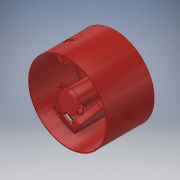
# Autodesk Inventor part: BottomPlatform
Saved by Autodesk Inventor 2019 (Build 230136000, 136)
## iProperties
Created: 2022-07-06
Part Number: BottomPlatform
Material: Generic
Document SubType Name: Modeling
Designer: zreik
Density: 1 g/cm^3
Appearance: Orange-Red
d104: 190.000 mm
Author: zreik
Autodesk Inventor part; units mm, degrees
ref_plane "XZ Plane" through (0, 0, 0) normal (0, 1, 0) x (-1, 0, 0)
ref_plane "XY Plane" through (0, 0, 0) normal (0, 0, 1) x (1, 0, 0)
sketch "Sketch1" plane through (0, 0, 0) normal (0, 0, 1) x (1, 0, 0)
  circle A0 centre (0, 0) radius 25
  line L0 (15, -5) -> (35, -5)
  line L1 (35, -5) -> (35, 5)
  line L2 (35, 5) -> (15, 5)
  line L3 (15, 5) -> (15, -5)
  line L4 (15, -5) -> (35, 5) construction
  line L5 (35, -5) -> (15, 5) construction
  point P0 (25, 0)
  dimension "d0" = 50
  dimension "d3" = 10
  dimension "d4" = 20
  dimension "d5" = 0
  constraints: 12 end point, 2 midpoint, 2 parallel, 1 coincident, 1 horizontal, 1 horizontal alignment, 1 perpendicular, 2 other
  measures "d3" distance of L0.end L1.end
  measures "d4" distance of L0.start L0.end
  measures "d5" vertical distance of point (0, 0) point (25, 0)
extrude "Extrusion1" add sketch "Sketch1" along normal mid plane 10 contours A0 L0 L3 L2 | L2 L3 L0 A0
extrude "Extrusion2" add sketch "Sketch1" along normal mid plane 10 contours A0 L0 L3 L2 | A0 L2 L1 L0 picked at (18.3333, 0)
chamfer "Chamfer1" distance 7 angle 30 1 edges at (35, 0, 5) measured on face at (34.5, 0, 5)
sketch "Sketch2" plane through (28, -5, 5) normal (0.5, 0, 0.8660254) x (0.8660254, 0, -0.5)
  line L0 (8.0829, 0) -> (0, 0)
  line L1 (0, 0) -> (0, 10)
  line L2 (0, 10) -> (8.0829, 10)
  line L3 (8.0829, 10) -> (8.0829, 0)
  line L4 (8.0829, 0) -> (0, 10) construction
  line L5 (0, 0) -> (8.0829, 10) construction
  line L6 (0, 10) -> (0, 0) projected
  line L7 (8.0829, 0) -> (8.0829, 10) projected
  line L8 (8.0829, 10) -> (0, 10) projected
  line L9 (0, 0) -> (8.0829, 0) projected
  point P0 (-21.7487, 5)
  point P1 (4.0415, 5)
  dimension "d11" = 0
  dimension "d12" = 0
  dimension "d13" = 0
  dimension "d14" = 0
  constraints: 12 end point, 2 midpoint, 2 parallel, 1 horizontal, 1 perpendicular
  measures "d11" distance between parallel lines of L1 L6
  measures "d12" distance between parallel lines of L7 L3
  measures "d13" distance between parallel lines of L8 L2
  measures "d14" distance between parallel lines of L9 L0
extrude "Extrusion3" add sketch "Sketch2" along normal blind 10
sketch "Sketch3" plane through (28, -5, 5) normal (-0.8660254, 0, 0.5) x (0.5, 0, 0.8660254)
  circle A0 centre (5, 5) radius 3.5
  line L0 (10, 10) -> (10, 0) projected
  line L1 (0, 10) -> (0, 0) projected
  line L2 (0, 0) -> (10, 0) projected
  line L3 (0, 10) -> (10, 10) projected
  point P0 (-18.3301, 5)
  dimension "d17" = 7
  dimension "d18" = 5
  dimension "d19" = 5
  dimension "d20" = 5
  dimension "d21" = 5
  constraints: 1 centre point
  measures "d17" diameter of A0
  measures "d18" distance from line of L0 A0.centre
  measures "d19" distance from line of L1 A0.centre
  measures "d20" distance from line of L2 A0.centre
  measures "d21" distance from line of L3 A0.centre
extrude "Extrusion5" cut sketch "Sketch3" against normal blind 3 contours A0
sketch "Sketch4" plane through (33.0981, 0, 7.8301) normal (-0.8660254, 0, 0.5) x (0.5, 0, 0.8660254)
  circle A0 centre (0, 0) radius 2.5
  circle A1 centre (0, 0) radius 3.5 projected
  point P0 (-23.3301, 0)
  dimension "d32" = 5
  constraints: 1 centre point, 1 concentric
  measures "d32" diameter of A0
extrude "Extrusion6" cut sketch "Sketch4" against normal through all contours A0
chamfer "Chamfer3" distance 5.5 angle 45 1 edges at (35, 0, -5)
sketch "Sketch5" plane through (35, -5, 0.9585) normal (0.8660254, 0, -0.5) x (-0.5, 0, -0.8660254)
  circle A0 centre (-5, 5) radius 3.5
  circle A1 centre (-5, 5) radius 2.5 projected
  point P0 (18.3301, 5)
  dimension "d35" = 7
  constraints: 1 centre point, 1 concentric
  measures "d35" diameter of A0
extrude "Extrusion7" cut sketch "Sketch5" against normal blind 3
pattern_circular "Circular Pattern1" count 3 over 360 about axis through (0, 0, 0) along (0, 0, 1) of "Extrusion3", "Extrusion2", "Chamfer1", "Extrusion5", "Extrusion6", "Extrusion7", "Chamfer3"
fillet "Fillet1" radius 2 12 edges at (-14, -24.2487, 5) (-14, 24.2487, 5) (28, 0, 5) (24.4949, -5, 0) (-7.9173, -23.7132, 0) (-16.5776, -18.7132, 0) (-16.5776, 18.7132, 0) (24.4949, 5, 0) (-7.9173, 23.7132, 0) (29.5, 0, -5) (-14.75, 25.5477, -5) (-14.75, -25.5477, -5)
fillet "Fillet2" radius 2 60 edges at (-22.5801, 29.1099, 11.6395) (-13.9199, 34.1099, 11.6395) (36.5, -5, 11.6395) (36.5, 5, 11.6395) (27.8453, -5, 5.2679) (26.4611, -5, 5) (24.8596, -5.413, 5) (12.5, -21.6506, 5) (-7.742, -24.2356, 5) (-8.9004, -25.4159, 5) (-9.5925, -26.6147, 5.2679) (-11.0642, -29.1638, 9.8301) (30.7887, -5, 9.8301) (-7.742, 24.2356, 5) (-8.9004, 25.4159, 5) (-9.5925, 26.6147, 5.2679) (-11.0642, 29.1638, 9.8301) (24.8596, 5.413, 5) (26.4611, 5, 5) (27.8453, 5, 5.2679) (30.7887, 5, 9.8301) (12.5, 21.6506, 5) (-17.1176, -18.8226, 5) (-17.5607, -20.4159, 5) (-18.2528, -21.6147, 5.2679) (-19.7245, -24.1638, 9.8301) (-17.1176, 18.8226, 5) (-17.5607, 20.4159, 5) (-18.2528, 21.6147, 5.2679) (-19.7245, 24.1638, 9.8301) (-25, 0, 5) (-7.742, -24.2356, -5) (-9.357, -26.2067, -5) (-10.3883, -27.9931, -4.8478) (-11.9413, -30.683, -1.9571) (24.8596, -5.413, -5) (27.3742, -5, -5) (29.4369, -5, -4.8478) (32.5429, -5, -1.9571) (12.5, -21.6506, -5) (-13.9199, -34.1099, 11.6395) (-22.5801, -29.1099, 11.6395) (-17.1176, 18.8226, -5) (-18.0172, 21.2067, -5) (-19.0486, 22.9931, -4.8478) (-20.6016, 25.683, -1.9571) (-17.1176, -18.8226, -5) (-18.0172, -21.2067, -5) (-19.0486, -22.9931, -4.8478) (-20.6016, -25.683, -1.9571) (-25, 0, -5) (24.8596, 5.413, -5) (27.3742, 5, -5) (29.4369, 5, -4.8478) (32.5429, 5, -1.9571) (-7.742, 24.2356, -5) (-9.357, 26.2067, -5) (-10.3883, 27.9931, -4.8478) (-11.9413, 30.683, -1.9571) (12.5, 21.6506, -5)
sketch "Sketch6" plane through (0, 0, -5) normal (0, 0, 1) x (1, 0, 0)
  line L0 (17, 16) -> (12, 16)
  line L1 (12, 16) -> (12, -16)
  line L2 (12, -16) -> (17, -16)
  line L3 (17, -16) -> (17, 16)
  point P0 (0, 0)
  dimension "d43" = 17
  dimension "d44" = 5
  dimension "d45" = 32
  dimension "d46" = 16
  constraints: 8 end point, 2 parallel, 1 horizontal, 1 perpendicular
  measures "d43" distance from line of L3 point (0, 0)
  measures "d44" distance between parallel lines of L1 L3
  measures "d45" distance between parallel lines of L2 L0
  measures "d46" distance from line of point (0, 0) L0
extrude "Extrusion8" add sketch "Sketch6" against normal blind 100
sketch "Sketch7" plane through (17, -16, -5) normal (1, 0, 0) x (0, 0, -1)
  line L0 (0, 10.037) -> (0, 0.5081) projected
  line L1 (0, 0) -> (100, 0) projected
  arc A0 (0, 10.037) -> (14.1552, 0) centre (14.1552, 15) ccw
  line L2 (14.1552, 0) -> (0, 0)
  line L3 (0, 0) -> (0, 10.037)
  line L4 (0, 32) -> (100, 32) projected
  ellipse E0 centre (-2, 21.963) end of major axis (0, 21.963) minor radius 0.5185 (0, 21.963) -> (-2, 22.4815) ccw projected
  line L5 (0, 31.4919) -> (0, 21.963) projected
  arc A1 (14.1552, 32) -> (0, 21.963) centre (14.1552, 17) ccw
  line L6 (0, 39) -> (0, 32) projected
  line L7 (14.1552, 32) -> (0, 32)
  line L8 (0, 32) -> (0, 21.963)
  line L9 (25, 0) -> (15, 0)
  line L10 (15, 0) -> (15, 32)
  line L11 (15, 32) -> (25, 32)
  line L12 (25, 32) -> (25, 0)
  line L13 (25, 30) -> (15, 30)
  line L14 (15, 30) -> (15, 2)
  line L15 (15, 2) -> (25, 2)
  line L16 (25, 2) -> (25, 30)
  line L17 (25, 26.5) -> (15, 26.5)
  line L18 (15, 26.5) -> (15, 5.5)
  line L19 (15, 5.5) -> (25, 5.5)
  line L20 (25, 5.5) -> (25, 26.5)
  point P0 (-5, 16)
  point P1 (0, 38.219)
  dimension "d49" = 0
  dimension "d50" = 15
  dimension "d53" = 0
  dimension "d54" = 15
  dimension "d57" = 10
  dimension "d58" = 15
  dimension "d59" = 0
  dimension "d60" = 0
  dimension "d61" = 2
  dimension "d62" = 2
  dimension "d70" = 21
  dimension "d71" = 5.5
  dimension "d72" = 5.5
  constraints: 32 end point, 6 parallel, 6 point on line, 5 perpendicular, 4 point on circle, 3 horizontal, 2 centre point, 2 collinear, 1 other
  measures "d49" horizontal distance of A0.centre L2.start
  measures "d50" radius of A0
  measures "d53" horizontal distance of L7.start A1.centre
  measures "d54" radius of A1
  measures "d57" distance between parallel lines of L10 L12
  measures "d58" distance between parallel lines of L0 L10
  measures "d59" distance between parallel lines of L12 L16
  measures "d60" distance between parallel lines of L10 L14
  measures "d61" distance between parallel lines of L9 L15
  measures "d62" distance between parallel lines of L4 L13
  measures "d70" distance between parallel lines of L19 L17
  measures "d71" distance between parallel lines of L4 L17
  measures "d72" distance between parallel lines of L9 L19
extrude "Extrusion9" cut sketch "Sketch7" against normal up to next contours A0 L1 L3 L0 | L4 A1 L5 L8
extrude "Extrusion10" cut sketch "Sketch7" against normal up to next contours L10 L19 L12 L15 | L10 L13 L12 L17
sketch "Sketch8" plane through (12, -16, -105) normal (0, -1, 0) x (1, 0, 0)
  circle A0 centre (2.5, 80) radius 1.5
  line L0 (0, 100) -> (0, 85.8448) projected
  line L1 (5, 75) -> (0, 75) projected
  point P0 (-12, 105)
  dimension "d65" = 2.5
  dimension "d66" = 3
  dimension "d67" = 5
  constraints: 1 centre point
  measures "d65" distance from line of L0 A0.centre
  measures "d66" diameter of A0
  measures "d67" distance from line of L1 A0.centre
extrude "Extrusion11" cut sketch "Sketch8" against normal blind 100
sketch "Sketch9" plane through (12, -16, -105) normal (-1, 0, 0) x (0, 0, 1)
  line L0 (0, 0) -> (0, 32) projected
  line L1 (50, 27) -> (0, 27)
  line L2 (0, 27) -> (0, 5)
  line L3 (0, 5) -> (50, 5)
  line L4 (50, 5) -> (50, 27)
  line L5 (85.8448, 0) -> (0, 0) projected
  line L6 (85.8448, 32) -> (0, 32) projected
  circle A0 centre (7.75, 2.5) radius 1.25
  circle A1 centre (15.75, 2.5) radius 1.25
  circle A2 centre (23.75, 2.5) radius 1.25
  circle A3 centre (31.75, 2.5) radius 1.25
  line L7 (77.9546, 16) -> (28.4498, 16) construction
  circle A4 centre (7.75, 29.5) radius 1.25
  circle A5 centre (15.75, 29.5) radius 1.25
  circle A6 centre (23.75, 29.5) radius 1.25
  circle A7 centre (31.75, 29.5) radius 1.25
  point P0 (105, 16)
  dimension "d73" = 22
  dimension "d74" = 5
  dimension "d75" = 5
  dimension "d76" = 50
  dimension "d77" = 0
  dimension "d78" = 0
  dimension "d79" = 0
  dimension "d80" = 8
  dimension "d81" = 2.5
  dimension "d82" = 8
  dimension "d83" = 8
  dimension "d84" = 2.5
  dimension "d85" = 2.5
  dimension "d86" = 2.5
  dimension "d87" = 7.75
  dimension "d88" = 2.5
  dimension "d89" = 16
  dimension "d90" = 16
  constraints: 10 end point, 8 centre point, 4 symmetric about line, 2 horizontal, 2 parallel, 1 perpendicular, 1 point on line, 4 other
  measures "d73" distance between parallel lines of L3 L1
  measures "d74" distance between parallel lines of L5 L3
  measures "d75" distance between parallel lines of L6 L1
  measures "d76" distance between parallel lines of L0 L4
  measures "d77" vertical distance of A1.centre A0.centre
  measures "d78" vertical distance of A2.centre A1.centre
  measures "d79" vertical distance of A3.centre A2.centre
  measures "d80" distance of A2.centre A3.centre
  measures "d81" diameter of A3
  measures "d82" distance of A1.centre A2.centre
  measures "d83" distance of A0.centre A1.centre
  measures "d84" diameter of A2
  measures "d85" diameter of A1
  measures "d86" diameter of A0
  measures "d87" distance from line of L0 A0.centre
  measures "d88" distance from line of L5 A0.centre
  measures "d89" distance between parallel lines of L5 L7
  measures "d90" distance between parallel lines of L6 L7
extrude "Extrusion12" cut sketch "Sketch9" against normal blind 100
pattern_circular "Circular Pattern2" count 3 over 360 about axis through (0, 0, 3) along (0, 0, 1) of "Extrusion8", "Extrusion9", "Extrusion10", "Extrusion11", "Extrusion12"
sketch "Sketch10" plane through (0, 0, -105) normal (0, 0, -1) x (-1, 0, 0)
  circle A0 centre (0, 0) radius 95
  circle A1 centre (0, 0) radius 85
  circle A2 centre (90, 0) radius 1.5
  circle A3 centre (-45, 77.9423) radius 1.5
  circle A4 centre (-45, -77.9423) radius 1.5
  arc A5 (5.9427, 22.219) -> (-22.2136, 5.963) centre (0, 0) ccw projected
  dimension "d98" = 190
  dimension "d99" = 170
  dimension "d100" = 3
  dimension "d103" = 360
  dimension "d206" = 90
  dimension "d207" = 0
  constraints: 5 centre point, 2 coincident, 1 concentric, 7 other
  measures "d98" diameter of A0
  measures "d99" diameter of A1
  measures "d100" diameter of A2
  measures "d206" distance of point (0, 0) A2.centre
  measures "d207" vertical distance of point (0, 0) A2.centre
extrude "Extrusion13" add sketch "Sketch10" along normal blind 5 contours A0 | A1
sketch "Sketch11" plane through (0, 0, -110) normal (0, 0, -1) x (-1, 0, 0)
  circle A0 centre (0, 0) radius 85
  circle A1 centre (0, 0) radius 83
  circle A2 centre (0, 0) radius 95 projected
  dimension "d107" = 2
  dimension "d108" = 10
  constraints: 2 centre point, 2 concentric
  measures "d107" radial gap between concentric circles of A0 A1
  measures "d108" radial gap between concentric circles of A2 A0
extrude "Extrusion14" add sketch "Sketch11" along normal blind 2 contours A0
ref_plane "Work Plane2" through (10.3564, -31.3827, -5) normal (0.5, -0.8660254, 0) x (0, 0, -1)
ref_plane "Work Plane1" through (5.3564, -22.7224, -5) normal (0.5, -0.8660254, 0) x (0, 0, -1)
sketch "Sketch12" plane through (10.3564, -31.3827, -5) normal (0.5, -0.8660254, 0) x (0, 0, -1)
  line L0 (20, 0) -> (100, 0)
  line L1 (100, 0) -> (100, 13.4449)
  line L2 (100, 13.4449) -> (20, 13.4449)
  line L3 (20, 13.4449) -> (20, 0)
  line L4 (100, 101.7224) -> (100, -88.2776) projected
  line L5 (14.1552, 13.4449) -> (100, 13.4449) projected
  line L6 (14.1552, 0) -> (100, 0) projected
  circle A0 centre (23, 6.7224) radius 1.5
  point P0 (-5, 6.7224)
  dimension "d112" = 0
  dimension "d113" = 80
  dimension "d114" = 0
  dimension "d115" = 0
  dimension "d116" = 3
  dimension "d117" = 6.7224
  dimension "d118" = 6.7224
  dimension "d119" = 3
  constraints: 8 end point, 2 parallel, 1 centre point, 1 horizontal, 1 perpendicular
  measures "d112" distance between parallel lines of L4 L1
  measures "d113" distance between parallel lines of L1 L3
  measures "d114" distance between parallel lines of L5 L2
  measures "d115" distance between parallel lines of L6 L0
  measures "d116" diameter of A0
  measures "d117" distance from line of L2 A0.centre
  measures "d118" distance from line of L0 A0.centre
  measures "d119" distance from line of L3 A0.centre
extrude "Extrusion15" add sketch "Sketch12" against normal blind 5
fillet "Fillet3" radius 5 2 edges at (20.75, -22.4952, -25) (9.1064, -29.2176, -25)
pattern_circular "Circular Pattern3" count 3 over 360 about axis through (0, 0, -110) along (0, 0, -1) of "Extrusion15", "Fillet3"
sketch "Sketch14" plane through (0, 0, 0) normal (1, 0, 0) x (0, 1, 0)
  line L0 (-150, -5) -> (150, -5)
  line L1 (150, -5) -> (150, -105)
  line L2 (150, -105) -> (-150, -105)
  line L3 (-150, -105) -> (-150, -5)
  line L4 (-5.963, -5) -> (-23, -5) projected
  line L5 (95, -105) -> (-95, -105) projected
  point P0 (0, 0)
  point P1 (-22.219, -5)
  dimension "d133" = 0
  dimension "d134" = 0
  dimension "d135" = 300
  dimension "d136" = 150
  constraints: 8 end point, 2 parallel, 1 horizontal, 1 perpendicular
  measures "d133" distance between parallel lines of L4 L0
  measures "d134" distance between parallel lines of L5 L2
  measures "d135" distance between parallel lines of L3 L1
  measures "d136" distance from line of point (0, 0) L3
extrude "Extrusion17" cut sketch "Sketch14" along normal through all both and the other way through all
ref_plane "Work Plane3" through (25, 0, 0) normal (1, 0, 0) x (0, 1, 0)
ref_plane "Work Plane5" through (37, 0, 0) normal (1, 0, 0) x (0, 1, 0)
sketch "Sketch15" plane through (37, 0, 0) normal (1, 0, 0) x (0, 1, 0)
  line L0 (-30, -30) -> (30, -30)
  line L1 (30, -30) -> (30, -105)
  line L2 (30, -105) -> (-30, -105)
  line L3 (-30, -105) -> (-30, -30)
  line L4 (95, -105) -> (-95, -105) projected
  point P0 (0, 0)
  dimension "d139" = 0
  dimension "d140" = 60
  dimension "d141" = 75
  dimension "d142" = 30
  constraints: 8 end point, 2 parallel, 1 horizontal, 1 perpendicular
  measures "d139" distance between parallel lines of L2 L4
  measures "d140" distance of L0.start L0.end
  measures "d141" distance of L2.end L0.start
  measures "d142" distance from line of point (0, 0) L3
extrude "Extrusion18" add sketch "Sketch15" along normal blind 50
ref_plane "Work Plane4" through (87, -30, -30) normal (0.5, 0, 0.8660254) x (0, -1, 0)
sketch "Sketch16" plane through (87, -30, -30) normal (0.5, 0, 0.8660254) x (0, -1, 0)
  line L0 (-14, -43.3013) -> (-46, -43.3013)
  line L1 (-46, -43.3013) -> (-46, -4.3013)
  line L2 (-46, -4.3013) -> (-14, -4.3013)
  line L3 (-14, -4.3013) -> (-14, -43.3013)
  line L4 (-60, 37.5) -> (-60, 0) projected
  line L5 (0, 0) -> (0, 37.5) projected
  line L6 (-60, 37.5) -> (0, 37.5) projected
  line L7 (0, -43.3013) -> (-60, -43.3013) projected
  point P0 (-30, -90.3442)
  dimension "d148" = 32
  dimension "d149" = 14
  dimension "d150" = 14
  dimension "d151" = 39
  dimension "d157" = 0
  constraints: 8 end point, 2 parallel, 1 horizontal, 1 perpendicular
  measures "d148" distance of L1.end L2.end
  measures "d149" distance between parallel lines of L4 L1
  measures "d150" distance between parallel lines of L5 L3
  measures "d151" distance of L0.end L1.end
  measures "d157" distance between parallel lines of L7 L0
extrude "Extrusion19" cut sketch "Sketch16" against normal up to surface surface through (37, 0, -67.5) normal (1, 0, 0)
sketch "Sketch18" plane through (87, 0, 0) normal (1, 0, 0) x (0, 0, -1)
  line L0 (105, 30) -> (105, -30) projected
  line L1 (105, 30) -> (30, 30)
  line L2 (30, 30) -> (30, -30)
  line L3 (30, -30) -> (105, -30)
  line L4 (105, -30) -> (105, 30)
  point P0 (0, 0)
  dimension "d192" = 75
  dimension "d193" = 60
  constraints: 8 end point, 2 parallel, 1 horizontal, 1 perpendicular
  measures "d192" distance of L2.end L3.end
  measures "d193" distance of L1.end L2.end
extrude "Extrusion23" add sketch "Sketch18" along normal up to surface round surface about axis through (0, 0, -105) along (0, 0, -1) radius 95 far side no
sketch "Sketch17" plane through (82.0333, -16, -30) normal (-0.8660254, 0, 0.5) x (0.5, 0, 0.8660254)
  circle A0 centre (-6.456, 2.5) radius 1.25
  circle A1 centre (-14.456, 2.5) radius 1.25
  circle A2 centre (-22.456, 2.5) radius 1.25
  line L0 (2.4833, 46) -> (2.4833, -14) projected
  line L1 (2.4833, -14) -> (-62.4686, -14) projected
  line L2 (0, 0) -> (-22.5167, 0) projected
  line L3 (12.9595, 16) -> (-31.8996, 16)
  circle A3 centre (-6.456, 29.5) radius 1.25
  circle A4 centre (-14.456, 29.5) radius 1.25
  circle A5 centre (-22.456, 29.5) radius 1.25
  line L4 (0, 32) -> (0, 0) projected
  line L5 (-10.206, 25.8) -> (-3.706, 25.8)
  line L6 (-3.706, 25.8) -> (-3.706, 6.2)
  line L7 (-3.706, 6.2) -> (-10.206, 6.2)
  line L8 (-10.206, 6.2) -> (-10.206, 25.8)
  line L9 (0, 25.8) -> (-3.706, 25.8)
  line L10 (-3.706, 25.8) -> (-3.706, 6.2)
  line L11 (-3.706, 6.2) -> (0, 6.2)
  line L12 (0, 6.2) -> (0, 25.8)
  point P0 (-15.0359, 16)
  dimension "d159" = 2.5
  dimension "d160" = 2.5
  dimension "d161" = 2.5
  dimension "d162" = 8
  dimension "d163" = 8
  dimension "d164" = 0
  dimension "d165" = 0
  dimension "d168" = 2.5
  dimension "d169" = 16
  dimension "d172" = 6.456
  dimension "d173" = 2.75
  dimension "d174" = 3.75
  dimension "d175" = 19.6
  dimension "d176" = 9.8
  dimension "d179" = 19.6
  dimension "d180" = 9.8
  dimension "d181" = 0
  dimension "d182" = 0
  constraints: 18 end point, 6 centre point, 4 parallel, 3 horizontal, 3 symmetric about line, 2 perpendicular, 3 other
  measures "d159" diameter of A0
  measures "d160" diameter of A1
  measures "d161" diameter of A2
  measures "d162" distance of A0.centre A1.centre
  measures "d163" distance of A1.centre A2.centre
  measures "d164" vertical distance of A2.centre A1.centre
  measures "d165" vertical distance of A1.centre A0.centre
  measures "d168" distance from line of L2 A0.centre
  measures "d169" distance between parallel lines of L2 L3
  measures "d172" distance from line of A0.centre L4
  measures "d173" distance from line of A0.centre L6
  measures "d174" distance from line of L8 A0.centre
  measures "d175" distance of L7.end L5.start
  measures "d176" distance between parallel lines of L3 L5
  measures "d179" distance of L9.end L10.end
  measures "d180" distance between parallel lines of L3 L11
  measures "d181" distance between parallel lines of L4 L12
  measures "d182" distance between parallel lines of L6 L10
sketch "Sketch20" plane through (0, 0, -105) normal (0, 0, 1) x (1, 0, 0)
  circle A0 centre (0, 0) radius 95
  circle A1 centre (0, 0) radius 93
  circle A2 centre (0, 0) radius 95 projected
  dimension "d203" = 186
  constraints: 2 centre point, 2 coincident, 1 concentric
  measures "d203" diameter of A1
extrude "Extrusion25" add sketch "Sketch20" along normal blind 110
extrude "Extrusion20" cut sketch "Sketch17" against normal up to next contours A0 | A1 | A2 | A3 | A4 | A5
extrude "Extrusion21" cut sketch "Sketch17" against normal up to next contours L6 L7 L8 L3 | L3 L8 L5 L6
extrude "Extrusion22" add sketch "Sketch17" along normal blind 3 contours L4 L11 L6 L3 | L3 L6 L9 L4
chamfer "Chamfer4" distance 40 angle 30 1 edges at (37, 23, -30) measured on face at (37, 23, -30.5)
chamfer "Chamfer5" distance 40 angle 30 1 edges at (37, -23, -30) measured on face at (37, -23, -30.5)
fillet "Fillet4" radius 2 8 edges at (60.094, -23, -30) (60.094, 23, -30) (37, 23, -70) (37, -23, -70) (74.0612, 30, -30) (74.0612, -30, -30) (48.547, 30, -50) (48.547, -30, -50)
pattern_circular "Circular Pattern4" count 3 over 360 about axis through (0, 0, -105) along (0, 0, -1) of "Fillet4", "Extrusion18", "Extrusion21", "Extrusion20", "Extrusion22", "Chamfer4", "Chamfer5", "Extrusion19", "Extrusion23"
sketch "Sketch19" plane through (0, 0, -5) normal (0, 0, -1) x (-1, 0, 0)
  circle A0 centre (0, 0) radius 22.5
  circle A1 centre (0, 0) radius 17.5
  dimension "d199" = 45
  dimension "d200" = 35
  constraints: 2 centre point, 2 coincident
  measures "d199" diameter of A0
  measures "d200" diameter of A1
extrude "Extrusion24" add sketch "Sketch19" along normal up to next
equation "\"d18\" = d19"
equation "\"d20\" = d21"
equation "\"d46\" = 0.5 * d45"
equation "\"d50\" = d54"
equation "\"d62\" = d61"
equation "\"d71\" = d72"
equation "\"d67\" = 0.5 * d57"
equation "\"d74\" = d75"
equation "\"d82\" = d80"
equation "\"d83\" = d82"
equation "\"d84\" = d81"
equation "\"d85\" = d84"
equation "\"d86\" = d85"
equation "\"d89\" = d90"
equation "\"d98\" = d104"
equation "\"d117\" = d118"
equation "\"d142\" = 0.5 * d140"
equation "\"d149\" = d150"
equation "\"d160\" = d159"
equation "\"d161\" = d160"
equation "\"d104\" = 190"
body "Solid1"
